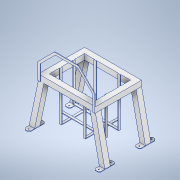
# Autodesk Inventor part: zweite_Ebene
Saved by Autodesk Inventor 2020 (Build 240168000, 168)
## iProperties
Created: 2020-05-27
Part Number: zweite_Ebene
Material: Aluminium 6061
Document SubType Name: Modeling
Designer: Chris
Density: 2.7 g/cm^3
Appearance: Aluminium - flach
Mass: 9688.38 g
Surface Area: 14689.5 cm^2
Volume: 3588.29 cm^3
Author: Chris
Autodesk Inventor part; units mm, degrees
ref_plane "YZ Plane" through (0, 0, 0) normal (1, 0, 0) x (0, 1, 0)
ref_plane "XZ Plane" through (0, 0, 0) normal (0, 1, 0) x (-1, 0, 0)
ref_plane "XY Plane" through (0, 0, 0) normal (0, 0, 1) x (1, 0, 0)
sketch "Skizze1" plane through (0, 0, 0) normal (0, 1, 0) x (-1, 0, 0)
  line L0 (0, 0) -> (420, 0)
  line L1 (420, 0) -> (420, -320)
  line L2 (420, -320) -> (0, -320)
  line L3 (0, -320) -> (0, 0)
  line L4 (0, 0) -> (-50, 0)
  line L5 (-50, 0) -> (-50, 50)
  line L6 (-50, 50) -> (0, 50)
  line L7 (0, 50) -> (0, 0)
  line L8 (-50, 50) -> (470, 50)
  line L9 (470, 50) -> (470, -370)
  line L10 (470, -370) -> (-50, -370)
  line L11 (-50, -370) -> (-50, 50)
  dimension "d0" = 420
  dimension "d1" = 320
  dimension "d2" = 50
  dimension "d3" = 50
  dimension "d4" = 520
  dimension "d5" = 420
  constraints: 24 end point, 6 parallel, 3 horizontal, 3 perpendicular
  measures "d0" distance of L1.end L2.end
  measures "d1" distance of L0.end L1.end
  measures "d2" distance of L5.end L6.end
  measures "d3" distance of L4.end L5.end
  measures "d4" distance of L9.end L10.end
  measures "d5" distance of L8.end L9.end
extrude "Extrusion1" add sketch "Skizze1" along normal blind 50
sketch "Skizze2" plane through (-470, 0, 50) normal (0, 0, 1) x (1, 0, 0)
  line L0 (520, 0) -> (0, 0) construction
  line L1 (0, 0) -> (0, -400) construction
  line L2 (0, -400) -> (-85, -400) construction
  line L3 (0, 0) -> (-85, -400)
  line L4 (-85, -400) -> (-35, -400)
  line L5 (-35, -400) -> (50, 0)
  line L6 (50, 0) -> (0, 0)
  line L7 (520, 0) -> (520, -400) construction
  line L8 (520, 0) -> (920, 0) construction
  line L9 (520, -400) -> (605, -400) construction
  line L10 (605, -400) -> (520, 0)
  line L11 (605, -400) -> (555, -400)
  line L12 (555, -400) -> (470, 0)
  line L13 (520, 0) -> (470, 0)
  dimension "d8" = 400
  dimension "d9" = 85
  dimension "d10" = 90
  dimension "d11" = 50
  dimension "d12" = 400
  dimension "d13" = 90
  dimension "d14" = 85
  dimension "d15" = 90
  dimension "d16" = 50
  constraints: 26 end point, 3 perpendicular, 3 point on line, 2 vertical, 1 collinear, 1 horizontal, 1 parallel
  measures "d8" distance of L0.end L1.end
  measures "d9" distance of L1.end L2.end
  measures "d10" angle of L1 L2
  measures "d11" distance of L2.end L4.end
  measures "d12" distance of L0.start L7.end
  measures "d13" angle of L7 L8
  measures "d14" distance of L7.end L9.end
  measures "d15" angle of L9 L7
  measures "d16" distance of L9.end L11.end
extrude "Extrusion2" add sketch "Skizze2" against normal blind 420
sketch "Skizze3" plane through (50, 50, 50) normal (1, 0, 0) x (0, 0, -1)
  line L0 (420, -50) -> (0, -50) construction
  line L1 (0, -50) -> (50, -50) construction
  line L2 (0, -450) -> (420, -450) projected
  line L3 (50, -50) -> (370, -50)
  line L4 (370, -50) -> (370, -450)
  line L5 (370, -450) -> (50, -450)
  line L6 (50, -450) -> (50, -50)
  dimension "d19" = 50
  dimension "d20" = 320
  constraints: 10 end point, 2 parallel, 1 collinear, 1 horizontal, 1 perpendicular, 1 point on line
  measures "d19" distance of L0.end L1.end
  measures "d20" distance of L4.end L5.end
extrude "Extrusion3" cut sketch "Skizze3" against normal mid plane 2000
shell "Wandung2" thickness 5 removed faces 4 at (-538.3333, -400, -336.6667) at (101.6667, -400, -336.6667) at (101.6667, -400, 33.3333) at (-538.3333, -400, 33.3333)
sketch "Skizze4" plane through (-555, -400, 50) normal (0, -1, 0) x (1, 0, 0)
  line L0 (0, 0) -> (0, -50) construction
  line L1 (0, 0) -> (0, 50) construction
  line L2 (0, 50) -> (50, 50)
  line L3 (50, 50) -> (50, -100)
  line L4 (50, -100) -> (0, -100)
  line L5 (0, -100) -> (0, 50)
  line L6 (85, 0) -> (605, 0) projected
  line L7 (345, 0) -> (345, -420)
  line L8 (555, -420) -> (135, -420) projected
  line L9 (85, -370) -> (85, -50) projected
  line L10 (85, -210) -> (605, -210)
  line L11 (605, 0) -> (605, -420) projected
  line L12 (690, 0) -> (690, -50) construction
  line L13 (690, 0) -> (690, 50) construction
  line L14 (690, 50) -> (640, 50)
  line L15 (640, 50) -> (640, -100)
  line L16 (640, -100) -> (690, -100)
  line L17 (690, -100) -> (690, 50)
  line L18 (0, -420) -> (0, -370) construction
  line L19 (0, -420) -> (0, -470) construction
  line L20 (0, -470) -> (50, -470)
  line L21 (50, -470) -> (50, -320)
  line L22 (50, -320) -> (0, -320)
  line L23 (0, -320) -> (0, -470)
  line L24 (640, -320) -> (690, -320)
  line L25 (640, -470) -> (640, -320)
  line L26 (690, -420) -> (690, -370) construction
  line L27 (690, -320) -> (690, -470)
  line L28 (690, -470) -> (640, -470)
  line L29 (690, -420) -> (690, -470) construction
  point P0 (555, -50)
  dimension "d25" = 50
  dimension "d26" = 50
  dimension "d27" = 150
  constraints: 50 end point, 18 symmetric about line, 4 midpoint, 2 parallel, 1 horizontal, 1 perpendicular, 1 vertical
  measures "d25" distance of L0.start L1.end
  measures "d26" distance of L3.end L4.end
  measures "d27" distance of L2.end L3.end
extrude "Extrusion4" add sketch "Skizze4" along normal blind 5 contours L2 L3 L4 L5 | L17 L16 L15 L14 | L23 L22 L21 L20 | L24 L27 L28 L25
chamfer "Fase1" distance 12.5 angle 45 16 edges at (-555, -402.5, 100) (-505, -402.5, 100) (85, -402.5, 100) (135, -402.5, 100) (85, -402.5, -270) (135, -402.5, -270) (-555, -402.5, -270) (-505, -402.5, -270) (-555, -402.5, -50) (-505, -402.5, -50) (-555, -402.5, -420) (-505, -402.5, -420) (85, -402.5, -50) (135, -402.5, -50) (85, -402.5, -420) (135, -402.5, -420)
sketch "Skizze5" plane through (-555, -405, 50) normal (0, -1, 0) x (1, 0, 0)
  line L0 (0, -370) -> (0, -420) projected
  line L1 (0, -395) -> (50, -395)
  line L2 (50, -370) -> (50, -420) projected
  line L3 (37.5, -320) -> (12.5, -320) projected
  line L4 (25, -320) -> (25, -340)
  circle A0 centre (25, -340) radius 4.5
  circle A1 centre (25, -450) radius 4.5
  line L5 (130.9509, -5) -> (559.0491, -5) projected
  line L6 (345, -5) -> (345, -420)
  line L7 (555, -420) -> (135, -420) projected
  line L8 (85, -420) -> (85, 0) projected
  line L9 (85, -210) -> (600, -210)
  line L10 (600, -5) -> (600, -415) projected
  circle A2 centre (25, -80) radius 4.5
  circle A3 centre (25, 30) radius 4.5
  circle A4 centre (665, -340) radius 4.5
  circle A5 centre (665, -450) radius 4.5
  circle A6 centre (665, -80) radius 4.5
  circle A7 centre (665, 30) radius 4.5
  point P0 (555, -50)
  dimension "d33" = 20
  dimension "d34" = 9
  constraints: 8 centre point, 8 end point, 7 midpoint, 7 symmetric about line, 1 coincident, 1 vertical, 7 other
  measures "d33" distance of L4.start L4.end
  measures "d34" diameter of A0
extrude "Extrusion5" cut sketch "Skizze5" against normal blind 5
sketch "Skizze6" plane through (0, 50, 0) normal (0, 1, 0) x (1, 0, 0)
  line L0 (-420, 320) -> (-470, 320) construction
  line L1 (-420, 320) -> (-330, 320) construction
  line L2 (-420, 320) -> (0, 320) construction
  line L3 (-420, 320) -> (-420, 230) construction
  line L4 (-420, 0) -> (-420, 320) construction
  line L5 (-330, 320) -> (-310, 320)
  line L6 (-310, 320) -> (-310, 315)
  line L7 (-310, 315) -> (-330, 315)
  line L8 (-330, 315) -> (-330, 320)
  line L9 (-420, 230) -> (-415, 230)
  line L10 (-415, 230) -> (-415, 210)
  line L11 (-415, 210) -> (-420, 210)
  line L12 (-420, 210) -> (-420, 230)
  line L13 (50, 370) -> (-470, 370) projected
  line L14 (-210, 370) -> (-210, -50)
  line L15 (-470, -50) -> (50, -50) projected
  line L16 (-470, 370) -> (-470, -50) projected
  line L17 (-470, 160) -> (236.5178, 160)
  line L18 (5, 325) -> (5, -5) projected
  line L19 (-330, 0) -> (-310, 0)
  line L20 (-310, 0) -> (-310, 5)
  line L21 (-310, 5) -> (-330, 5)
  line L22 (-330, 5) -> (-330, 0)
  line L23 (-420, 90) -> (-415, 90)
  line L24 (-415, 90) -> (-415, 110)
  line L25 (-415, 110) -> (-420, 110)
  line L26 (-420, 110) -> (-420, 90)
  line L27 (-90, 320) -> (-110, 320)
  line L28 (-110, 320) -> (-110, 315)
  line L29 (-110, 315) -> (-90, 315)
  line L30 (-90, 315) -> (-90, 320)
  line L31 (0, 230) -> (-5, 230)
  line L32 (-5, 230) -> (-5, 210)
  line L33 (-5, 210) -> (0, 210)
  line L34 (0, 210) -> (0, 230)
  line L35 (0, 90) -> (-5, 90)
  line L36 (-5, 110) -> (0, 110)
  line L37 (0, 110) -> (0, 90)
  line L38 (-5, 90) -> (-5, 110)
  line L39 (-90, 5) -> (-90, 0)
  line L40 (-90, 0) -> (-110, 0)
  line L41 (-110, 0) -> (-110, 5)
  line L42 (-110, 5) -> (-90, 5)
  point P0 (0, 0)
  dimension "d37" = 90
  dimension "d38" = 90
  dimension "d39" = 20
  dimension "d40" = 5
  dimension "d41" = 5
  dimension "d42" = 20
  constraints: 72 end point, 24 symmetric about line, 4 parallel, 3 midpoint, 3 perpendicular, 2 horizontal, 2 point on line
  measures "d37" distance of L0.start L1.end
  measures "d38" distance of L0.start L3.end
  measures "d39" distance of L6.end L7.end
  measures "d40" distance of L5.end L6.end
  measures "d41" distance of L10.end L11.end
  measures "d42" distance of L9.end L10.end
extrude "Extrusion6" add sketch "Skizze6" against normal blind 345 contours L5 L6 L7 L8 | L9 L10 L11 L12 | L22 L21 L20 L19 | L26 L25 L24 L23 | L30 L29 L28 L27 | L34 L33 L32 L31 | L35 L38 L36 L37 | L39 L40 L41 L42
sketch "Skizze7" plane through (-415, -295, -90) normal (0, 0, 1) x (1, 0, 0)
  line L0 (-5, 0) -> (0, 0) projected
  line L1 (0, 0) -> (-5, 0)
  line L2 (-5, 0) -> (-5, 5)
  line L3 (-5, 5) -> (0, 5)
  line L4 (0, 5) -> (0, 0)
  line L5 (409.2958, 0) -> (419.1788, 0)
  line L6 (419.1788, 0) -> (419.1788, 5)
  line L7 (419.1788, 5) -> (409.2958, 5)
  line L8 (409.2958, 5) -> (409.2958, 0)
  point P0 (415, 295)
  dimension "d45" = 5
  dimension "d46" = 5
  dimension "d47" = 5
  constraints: 16 end point, 4 parallel, 2 horizontal, 2 perpendicular, 1 point on line
  measures "d45" distance of L2.end L3.end
  measures "d46" distance of L1.end L2.end
  measures "d47" distance of L6.end L5.end
extrude "Extrusion7" cut sketch "Skizze7" against normal blind 345
sketch "Skizze8" plane through (-420, -290, -90) normal (0, -1, 0) x (1, 0, 0)
  line L0 (0, 90) -> (0, 0) projected
  line L1 (0, 0) -> (420, 0)
  line L2 (420, 0) -> (420, -20)
  line L3 (420, -20) -> (0, -20)
  line L4 (0, -20) -> (0, 0)
  line L5 (0, -120) -> (0, -140) projected
  line L6 (420, -140) -> (420, -120) projected
  line L7 (0, -120) -> (420, -120)
  line L8 (420, -120) -> (420, -140)
  line L9 (420, -140) -> (0, -140)
  line L10 (0, -140) -> (0, -120)
  point P0 (420, 90)
  constraints: 16 end point, 4 parallel, 2 horizontal, 2 perpendicular
extrude "Extrusion8" add sketch "Skizze8" along normal blind 5
sketch "Skizze9" plane through (0, -295, 0) normal (0, -1, 0) x (1, 0, 0)
  line L0 (-330, -320) -> (-310, -320) projected
  line L1 (-330, 0) -> (-310, 0)
  line L2 (-310, 0) -> (-310, -320)
  line L3 (-310, -320) -> (-330, -320)
  line L4 (-330, -320) -> (-330, 0)
  line L5 (-90, 0) -> (-110, 0) projected
  line L6 (-89.9794, -320) -> (-110, -320)
  line L7 (-110, -320) -> (-110, 0)
  line L8 (-110, 0) -> (-89.9794, 0)
  line L9 (-89.9794, 0) -> (-89.9794, -320)
  point P0 (0, 0)
  constraints: 16 end point, 4 parallel, 2 horizontal, 2 perpendicular, 1 point on line
extrude "Extrusion9" add sketch "Skizze9" along normal blind 5
sketch "Skizze10" plane through (-470, 50, 50) normal (0, 0, 1) x (1, 0, 0)
  line L0 (520, -50) -> (470, -50) projected
  line L1 (520, -50) -> (500, -50)
  line L2 (500, -50) -> (500, 100)
  line L3 (500, 100) -> (520, 100)
  line L4 (520, 100) -> (520, -50)
  line L5 (0.1359, -50) -> (20.1359, -50)
  line L6 (20.1359, -50) -> (20.1359, 100)
  line L7 (20.1359, 100) -> (0.1359, 100)
  line L8 (0.1359, 100) -> (0.1359, -50)
  line L9 (0.1359, 100) -> (280.1125, 379.9766) construction
  line L10 (0.1359, 100) -> (396.0827, 100) construction
  line L11 (520, 100) -> (260.068, 359.932) construction
  line L12 (520, 100) -> (887.5994, 100) construction
  line L13 (360, 0) -> (160, 0) construction
  line L14 (260, 0) -> (260, 250) construction
  line L15 (260, 0) -> (510, 0) construction
  line L16 (260, 250) -> (150.1359, 250) construction
  line L17 (260, 250) -> (370, 250) construction
  line L18 (0.1359, 100) -> (150.1359, 250)
  line L19 (150.1359, 250) -> (370, 250)
  line L20 (370, 250) -> (520, 100)
  line L21 (370, 250) -> (355.8579, 235.8579) construction
  line L22 (150.1359, 250) -> (164.2781, 235.8579) construction
  line L23 (370, 250) -> (520, 100)
  line L24 (520, 100) -> (505.8579, 85.8579)
  line L25 (505.8579, 85.8579) -> (355.8579, 235.8579)
  line L26 (355.8579, 235.8579) -> (370, 250)
  line L27 (370, 250) -> (150.1359, 250)
  line L28 (150.1359, 250) -> (150.1359, 230)
  line L29 (150.1359, 230) -> (370, 230)
  line L30 (370, 230) -> (370, 250)
  line L31 (150.1359, 250) -> (0.1359, 100)
  line L32 (0.1359, 100) -> (14.2781, 85.8579)
  line L33 (14.2781, 85.8579) -> (164.2781, 235.8579)
  line L34 (164.2781, 235.8579) -> (150.1359, 250)
  point P0 (20.1359, 91.7157)
  point P1 (158.4202, 230)
  point P2 (361.7157, 230)
  point P3 (500, 91.7157)
  dimension "d54" = 20
  dimension "d55" = 150
  dimension "d56" = 20
  dimension "d57" = 150
  dimension "d58" = 45
  dimension "d59" = 135
  dimension "d60" = 250
  dimension "d61" = 90
  dimension "d62" = 20
  dimension "d63" = 20
  dimension "d64" = 20
  dimension "d65" = 20
  dimension "d66" = 20
  constraints: 66 end point, 10 parallel, 10 perpendicular, 5 horizontal, 5 point on line, 3 collinear, 3 equal length, 1 midpoint, 1 vertical
  measures "d54" distance of L2.end L3.end
  measures "d55" distance of L1.end L2.end
  measures "d56" distance of L7.end L6.end
  measures "d57" distance of L6.end L5.end
  measures "d58" angle of L10 L9
  measures "d59" angle of L12 L11
  measures "d60" distance of L14.start L14.end
  measures "d61" angle of L15 L14
  measures "d62" distance of L17.end L21.end
  measures "d63" distance of L18.end L22.end
  measures "d64" distance of L3.end L24.end
  measures "d65" distance of L28.end L18.end
  measures "d66" distance of L32.end L7.end
extrude "Extrusion10" add sketch "Skizze10" along normal blind 5
